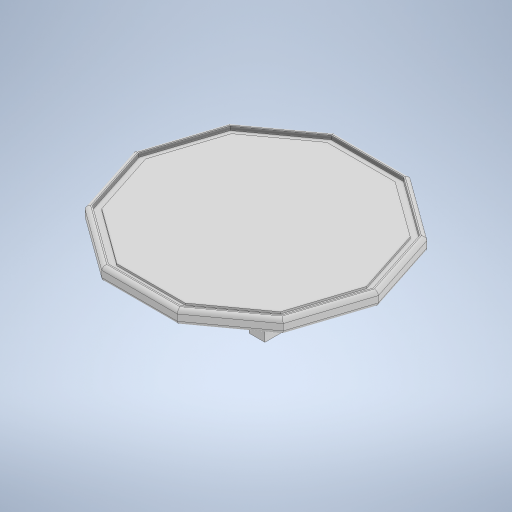
# Autodesk Inventor part: OV-PAM_n_10_bottom
Saved by Autodesk Inventor 2024 (Build 280153000, 153)
## iProperties
Created: 2023-08-31
Part Number: OV-PAM_n_10_bottom
Material: 일반
Document SubType Name: Modeling
Designer: jsw
Density: 1 g/cm^3
Appearance: 기본값
Author: jsw
Autodesk Inventor part; units mm, degrees
ref_plane "YZ Plane" through (0, 0, 0) normal (1, 0, 0) x (0, 1, 0)
ref_plane "XZ Plane" through (0, 0, 0) normal (0, 1, 0) x (-1, 0, 0)
ref_plane "XY Plane" through (0, 0, 0) normal (0, 0, 1) x (1, 0, 0)
sketch "스케치1" plane through (0, 0, 0) normal (0, 1, 0) x (-1, 0, 0)
  line L0 (-10.9012, 33.5504) -> (10.9012, 33.5504)
  line L1 (10.9012, 33.5504) -> (28.5397, 20.7353)
  line L2 (28.5397, 20.7353) -> (35.277, 0)
  line L3 (35.277, 0) -> (28.5397, -20.7353)
  line L4 (28.5397, -20.7353) -> (10.9012, -33.5504)
  line L5 (10.9012, -33.5504) -> (-10.9012, -33.5504)
  line L6 (-10.9012, -33.5504) -> (-28.5397, -20.7353)
  line L7 (-28.5397, -20.7353) -> (-35.277, 0)
  line L8 (-35.277, 0) -> (-28.5397, 20.7353)
  line L9 (-28.5397, 20.7353) -> (-10.9012, 33.5504)
  line L10 (11.9409, -36.7504) -> (-11.9409, -36.7504)
  line L11 (-11.9409, -36.7504) -> (-31.2618, -22.713)
  line L12 (-31.2618, -22.713) -> (-38.6417, 0)
  line L13 (-38.6417, 0) -> (-31.2618, 22.713)
  line L14 (-31.2618, 22.713) -> (-11.9409, 36.7504)
  line L15 (-11.9409, 36.7504) -> (11.9409, 36.7504)
  line L16 (11.9409, 36.7504) -> (31.2618, 22.713)
  line L17 (31.2618, 22.713) -> (38.6417, 0)
  line L18 (38.6417, 0) -> (31.2618, -22.713)
  line L19 (31.2618, -22.713) -> (11.9409, -36.7504)
  point P0 (0, 0)
  point P1 (0, 0)
  point P2 (0, 0)
  dimension "d0" = 70.554
  dimension "d1" = 3.2
  constraints: 40 end point, 2 coincident, 2 horizontal, 42 other
  measures "d0" distance of L7.end L2.end
  measures "d1" distance between parallel lines of L3 L18
extrude "돌출1" add sketch "스케치1" along normal blind 4.4 contours L0 L1 L2 L3 L4 L5 L6 L7 L8 L9 | L10 L11 L12 L13 L14 L15 L16 L17 L18 L19
sketch "스케치2" plane through (0, 4.4, 0) normal (0, 1, 0) x (1, 0, 0)
  line L0 (-11.4211, 35.1504) -> (11.4211, 35.1504)
  line L1 (11.4211, 35.1504) -> (29.9007, 21.7242)
  line L2 (29.9007, 21.7242) -> (36.9593, 0)
  line L3 (36.9593, 0) -> (29.9007, -21.7242)
  line L4 (29.9007, -21.7242) -> (11.4211, -35.1504)
  line L5 (11.4211, -35.1504) -> (-11.4211, -35.1504)
  line L6 (-11.4211, -35.1504) -> (-29.9007, -21.7242)
  line L7 (-29.9007, -21.7242) -> (-36.9593, 0)
  line L8 (-36.9593, 0) -> (-29.9007, 21.7242)
  line L9 (-29.9007, 21.7242) -> (-11.4211, 35.1504)
  line L10 (-31.2618, 22.713) -> (-38.6417, 0) projected
  point P0 (0, 0)
  point P1 (0, 0)
  dimension "d4" = 1.6
  constraints: 20 end point, 1 coincident, 1 horizontal, 21 other
  measures "d4" distance between parallel lines of L8 L10
extrude "돌출2" cut sketch "스케치2" against normal blind 1.2
sketch "스케치3" plane through (0, 3.2, 0) normal (0, 1, 0) x (1, 0, 0)
  line L0 (-10.7712, 33.1504) -> (10.7712, 33.1504)
  line L1 (10.7712, 33.1504) -> (28.1994, 20.4881)
  line L2 (28.1994, 20.4881) -> (34.8564, 0)
  line L3 (34.8564, 0) -> (28.1994, -20.4881)
  line L4 (28.1994, -20.4881) -> (10.7712, -33.1504)
  line L5 (10.7712, -33.1504) -> (-10.7712, -33.1504)
  line L6 (-10.7712, -33.1504) -> (-28.1994, -20.4881)
  line L7 (-28.1994, -20.4881) -> (-34.8564, 0)
  line L8 (-34.8564, 0) -> (-28.1994, 20.4881)
  line L9 (-28.1994, 20.4881) -> (-10.7712, 33.1504)
  line L10 (-29.9007, 21.7242) -> (-11.4211, 35.1504) projected
  point P0 (0, 0)
  point P1 (0, 0)
  dimension "d7" = 2
  constraints: 20 end point, 1 coincident, 1 horizontal, 21 other
  measures "d7" distance between parallel lines of L10 L9
extrude "돌출3" add sketch "스케치3" along normal blind 0.6
fillet "모깎기1" radius 1.2 20 edges at (0, 4.4, 36.7504) (0, 0, 36.7504) (-21.6014, 4.4, 29.7317) (-21.6014, 0, 29.7317) (-34.9517, 4.4, 11.3565) (-34.9517, 4.4, -11.3565) (-21.6014, 4.4, -29.7317) (0, 4.4, -36.7504) (21.6014, 4.4, -29.7317) (34.9517, 4.4, -11.3565) (34.9517, 4.4, 11.3565) (21.6014, 4.4, 29.7317) (21.6014, 0, -29.7317) (0, 0, -36.7504) (-21.6014, 0, -29.7317) (-34.9517, 0, -11.3565) (-34.9517, 0, 11.3565) (34.9517, 0, -11.3565) (34.9517, 0, 11.3565) (21.6014, 0, 29.7317)
sketch "스케치10" plane through (0, 0, 0) normal (0, -1, 0) x (1, 0, 0)
  line L0 (10.3, 12.5) -> (15.3, 12.5)
  line L1 (15.3, 12.5) -> (15.3, -12.5)
  line L2 (15.3, -12.5) -> (10.3, -12.5)
  line L3 (10.3, -12.5) -> (10.3, 12.5)
  line L4 (10.3, 12.5) -> (15.3, -12.5) construction
  line L5 (15.3, 12.5) -> (10.3, -12.5) construction
  line L6 (0, 0) -> (0, -7.1527)
  line L7 (-10.3, 12.5) -> (-15.3, 12.5)
  line L8 (-15.3, 12.5) -> (-15.3, -12.5)
  line L9 (-15.3, -12.5) -> (-10.3, -12.5)
  line L10 (-10.3, -12.5) -> (-10.3, 12.5)
  line L11 (-10.3, 12.5) -> (-15.3, -12.5) construction
  line L12 (-15.3, 12.5) -> (-10.3, -12.5) construction
  point P0 (12.8, 0)
  point P1 (-12.8, 0)
  dimension "d50" = 5
  dimension "d51" = 25
  dimension "d52" = 10.3
  constraints: 26 end point, 5 symmetric about line, 2 midpoint, 2 parallel, 1 horizontal, 1 horizontal alignment, 1 perpendicular, 1 vertical
  measures "d50" distance of L1.end L2.end
  measures "d51" distance of L0.end L1.end
  measures "d52" distance from line of L3 L6.start
extrude "돌출7" add sketch "스케치10" along normal blind 15
sketch "스케치11" plane through (15.3, 0, 12.5) normal (1, 0, 0) x (0, 0, -1)
  circle A0 centre (7.5, -7.5) radius 1.25
  line L0 (-9.4714, 0) -> (12.5, 0) projected
  line L1 (12.5, 1.2) -> (12.5, 3.2) projected
  line L2 (12.5, 0) -> (12.5, -3.4496)
  circle A1 centre (17.5, -7.5) radius 1.25
  point P0 (12.5, 2.2)
  dimension "d55" = 2.5
  dimension "d56" = 7.5
  dimension "d57" = 5
  constraints: 2 centre point, 2 end point, 1 midpoint, 1 symmetric about line, 1 vertical, 1 other
  measures "d55" diameter of A0
  measures "d56" distance from line of A0.centre L0
  measures "d57" horizontal distance of point (12.5, 2.2) A0.centre
extrude "돌출8" cut sketch "스케치11" against normal up to surface (30.6 mm away)
equation "\"d38\" = 55deg"
